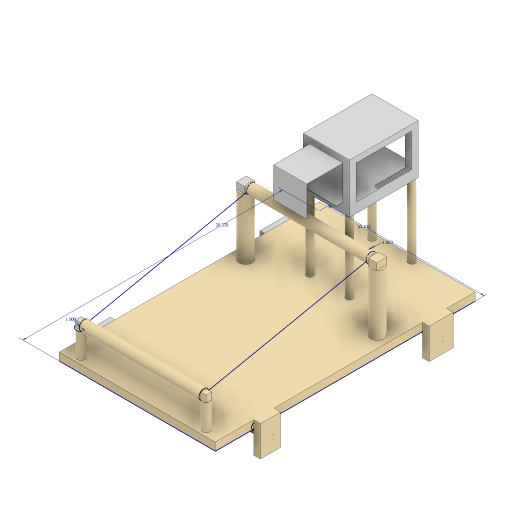
# Autodesk Inventor part: neha_chassis
Saved by Autodesk Inventor 2024 (Build 280153000, 153)
## iProperties
Created: 2023-06-06
Part Number: neha_chassis
Material: Generic
Document SubType Name: Modeling
Designer: ANIRUDH
Density: 1 g/cm^3
Appearance: Default
Author: ANIRUDH
Autodesk Inventor part; units mm, degrees
ref_plane "YZ Plane" through (0, 0, 0) normal (1, 0, 0) x (0, 1, 0)
ref_plane "XZ Plane" through (0, 0, 0) normal (0, 1, 0) x (-1, 0, 0)
sketch "Sketch1" plane through (0, 0, 0) normal (0, 1, 0) x (-1, 0, 0)
  line L0 (-300, -500) -> (300, -500)
  line L1 (300, -500) -> (300, 500)
  line L2 (300, 500) -> (-300, 500)
  line L3 (-300, 500) -> (-300, -500)
  line L4 (-300, -500) -> (300, 500) construction
  line L5 (300, -500) -> (-300, 500) construction
  circle A0 centre (76.2, -479.4561) radius 12.7
  circle A1 centre (-76.2, -479.4561) radius 12.7
  circle A2 centre (76.2, -479.4561) radius 12.7
  point P0 (0, 0)
  dimension "d14" = 600
  dimension "d15" = 1000
  dimension "d24" = 25.4
  constraints: 12 end point, 3 centre point, 2 midpoint, 2 parallel, 1 coincident, 1 concentric, 1 horizontal, 1 perpendicular
  measures "d14" distance of L0.start L0.end
  measures "d15" distance of L0.end L1.end
  measures "d24" diameter of A0
extrude "Extrusion1" add sketch "Sketch1" along normal blind 30 contours L3 L2 L1 L0 | A0 | A1
sketch "Sketch2" plane through (0, 30, 0) normal (0, 1, 0) x (1, 0, 0)
  line L0 (-300, 500) -> (-300, -500) projected
  circle A0 centre (-240.3274, -476.0112) radius 15
  circle A1 centre (241.3, -476.0112) radius 15
  line L1 (300, -500) -> (300, 500) projected
  line L2 (-240.3274, -476.0112) -> (-240.3274, 285.9888)
  line L3 (241.3, -476.0112) -> (241.3, 278.78)
  point P0 (0, 0)
  dimension "d6" = 30
  dimension "d7" = 30
  dimension "d19" = 762
  constraints: 4 end point, 2 centre point, 1 parallel, 1 vertical
  measures "d6" diameter of A0
  measures "d7" diameter of A1
  measures "d19" distance of L2.start L2.end
extrude "Extrusion2" add sketch "Sketch2" along normal blind 100
sketch "Sketch3" plane through (0, 30, 0) normal (0, 1, 0) x (1, 0, 0)
  line L0 (-300, 500) -> (-300, -500) projected
  circle A0 centre (-251.2271, 168.147) radius 25
  circle A1 centre (256.3, 168.147) radius 25
  circle A2 centre (241.3, -476.0112) radius 15 projected
  circle A3 centre (-240.3274, -476.0112) radius 15 projected
  line L1 (269, 155.447) -> (243.6, 180.847) construction
  line L2 (243.6, 155.447) -> (269, 180.847) construction
  point P0 (0, 0)
  dimension "d11" = 50
  dimension "d40" = 25.4
  dimension "d41" = 25.4
  constraints: 4 end point, 2 centre point, 2 midpoint
  measures "d11" diameter of A1
  measures "d40" distance of L1.end L2.end
  measures "d41" distance of L2.start L1.end
extrude "Extrusion3" add sketch "Sketch3" along normal blind 233.807 contours A0 | A1
ref_plane "Work Plane1" through (300, 30, 500) normal (1, 0, 0) x (0, 0, -1)
extrude "Extrusion4" add sketch "Sketch1" along normal blind 309.3974 contours A0 | A1
sketch "Sketch4" plane through (0, 30, 0) normal (0, 1, 0) x (1, 0, 0)
  circle A0 centre (-251.2271, 168.147) radius 25 projected
  circle A1 centre (256.3, 168.147) radius 25 projected
  circle A2 centre (-76.2, 479.4561) radius 12.7 projected
  circle A3 centre (76.2, 479.4561) radius 12.7 projected
  line L0 (76.2, 479.4561) -> (251.876, 479.4561) construction
  circle A4 centre (-76.2, 240.5293) radius 12.7
  circle A5 centre (76.2, 240.5293) radius 12.7
  point P0 (0, 0)
  dimension "d28" = 25.4
  constraints: 2 centre point, 2 end point, 1 horizontal
  measures "d28" diameter of A4
extrude "Extrusion5" add sketch "Sketch4" along normal blind 279.4 contours A4 | A5
sketch "Sketch5" plane through (-76.2, 309.3974, -479.4561) normal (0, 1, 0) x (1, 0, 0)
  line L0 (-14.696, 14.9952) -> (168.2208, 14.9952)
  line L1 (168.2208, 14.9952) -> (168.2208, -255.5835)
  line L2 (168.2208, -255.5835) -> (-14.696, -255.5835)
  line L3 (-14.696, -255.5835) -> (-14.696, 14.9952)
  point P0 (76.2, -479.4561)
  constraints: 8 end point, 2 parallel, 1 horizontal, 1 perpendicular
extrude "Extrusion6" [suppressed]
sketch "Sketch6" plane through (-76.2, 309.3974, -479.4561) normal (0, 1, 0) x (1, 0, 0)
  line L0 (-12.7, 12.7) -> (165.1, 12.7)
  line L1 (165.1, 12.7) -> (165.1, -251.6267)
  line L2 (165.1, -251.6267) -> (-12.7, -251.6267)
  line L3 (-12.7, -251.6267) -> (-12.7, 12.7)
  point P0 (76.2, -479.4561)
  constraints: 8 end point, 2 parallel, 1 horizontal, 1 perpendicular
extrude "Extrusion7" add sketch "Sketch6" along normal blind 12.7
sketch "Sketch7" plane through (300, 0, 500) normal (1, 0, 0) x (0, 0, -1)
  circle A0 centre (149.4368, 9.9643) radius 11.0201
  circle A1 centre (832.4462, 9.9643) radius 9.0585
  point P0 (500, 0)
  constraints: 2 centre point
sketch "Sketch8" plane through (300, 0, 500) normal (1, 0, 0) x (0, 0, -1)
  line L0 (1000, 30) -> (0, 30) projected
  line L1 (148.2506, 30) -> (226.2157, 30)
  line L2 (226.2157, 30) -> (226.2157, -87.9373)
  line L3 (226.2157, -87.9373) -> (148.2506, -87.9373)
  line L4 (148.2506, -87.9373) -> (148.2506, 30)
  line L5 (797.3552, 30) -> (889.8254, 30)
  line L6 (889.8254, 30) -> (889.8254, -87.9373)
  line L7 (889.8254, -87.9373) -> (797.3552, -87.9373)
  line L8 (797.3552, -87.9373) -> (797.3552, 30)
  point P0 (500, 0)
  point P1 (226.2157, 30)
  constraints: 16 end point, 4 parallel, 3 point on line, 2 horizontal, 2 perpendicular
extrude "Extrusion8" add sketch "Sketch8" along normal blind 25.4
sketch "Sketch9" plane through (-300, 0, -500) normal (-1, 0, 0) x (0, 0, 1)
  line L0 (202.6448, -87.9373) -> (110.1746, -87.9373) projected
  line L1 (108.3615, 22.6643) -> (202.6448, 22.6643)
  line L2 (202.6448, 22.6643) -> (202.6448, -87.9373)
  line L3 (202.6448, -87.9373) -> (108.3615, -87.9373)
  line L4 (108.3615, -87.9373) -> (108.3615, 22.6643)
  line L5 (777.4106, 22.6643) -> (851.7494, 22.6643)
  line L6 (851.7494, 22.6643) -> (851.7494, -87.9373)
  line L7 (851.7494, -87.9373) -> (777.4106, -87.9373)
  line L8 (777.4106, -87.9373) -> (777.4106, 22.6643)
  circle A0 centre (142.8112, -48.0482) radius 9.2452
  point P0 (500, 0)
  constraints: 16 end point, 4 parallel, 2 horizontal, 2 perpendicular, 2 point on line, 1 centre point
extrude "Extrusion9" add sketch "Sketch9" along normal blind 25.4 contours L0 L3 L4 L1 L2 | L5 L6 L7 L8 | A0
sketch "Sketch10" plane through (-325.4, 0, -500) normal (-1, 0, 0) x (0, 0, 1)
  circle A0 centre (151.8769, -29.9168) radius 8.1086
  circle A1 centre (802.7946, -29.9168) radius 7.2526
  point P0 (500, 0)
  constraints: 2 centre point
hole "Hole1" at (-325.4, -29.9168, -348.1231) at (-325.4, -29.9168, 302.7946) direction (1, 0, 0) diameter 1.4249 end through all thread size "1-64 UNC" class "2B" standard "ANSI Unified Screw Threads"
sketch "Sketch11" plane through (-325.4, 0, -500) normal (-1, 0, 0) x (0, 0, 1)
  circle A0 centre (148.2506, -46.2351) radius 11.6098
  circle A1 centre (802.7946, -46.2351) radius 11.6316
  point P0 (500, 0)
  constraints: 2 centre point
hole "Hole2" at (-325.4, -46.2351, -351.7494) at (-325.4, -46.2351, 302.7946) direction (1, 0, 0) diameter 1.4249 end through all thread size "1-64 UNC" class "2B" standard "ANSI Unified Screw Threads"
sketch "Sketch12" plane through (-325.4, 0, -500) normal (-1, 0, 0) x (0, 0, 1)
  circle A0 centre (151.8769, -29.9168) radius 0.7125 projected
  circle A1 centre (148.2506, -46.2351) radius 0.7125 projected
  circle A2 centre (151.8769, -29.9168) radius 16.7163
  circle A3 centre (813.6734, -46.6332) radius 18.1314
  point P0 (500, 0)
  constraints: 1 centre point, 1 coincident, 3 other
hole "Hole3" at (-325.4, -29.9168, -348.1231) at (-325.4, -46.6332, 313.6734) direction (1, 0, 0) diameter 1.4249 end through all thread size "1-64 UNC" class "2B" standard "ANSI Unified Screw Threads"
sketch "Sketch13" plane through (-251.2271, 263.807, -168.147) normal (0, 1, 0) x (1, 0, 0)
  circle A0 centre (0, 0) radius 25 projected
  line L0 (-16.0914, -19.1329) -> (16.0914, -19.1329)
  line L1 (16.0914, -19.1329) -> (16.0914, 19.1329)
  line L2 (16.0914, 19.1329) -> (-16.0914, 19.1329)
  line L3 (-16.0914, 19.1329) -> (-16.0914, -19.1329)
  line L4 (-16.0914, -19.1329) -> (16.0914, 19.1329) construction
  line L5 (16.0914, -19.1329) -> (-16.0914, 19.1329) construction
  circle A1 centre (507.5271, 0) radius 25 projected
  line L6 (482.5271, 0) -> (507.5271, 0)
  line L7 (491.4357, -19.1329) -> (523.6185, -19.1329)
  line L8 (523.6185, -19.1329) -> (523.6185, 19.1329)
  line L9 (523.6185, 19.1329) -> (491.4357, 19.1329)
  line L10 (491.4357, 19.1329) -> (491.4357, -19.1329)
  line L11 (491.4357, -19.1329) -> (523.6185, 19.1329) construction
  line L12 (523.6185, -19.1329) -> (491.4357, 19.1329) construction
  point P0 (251.2271, -168.147)
  constraints: 26 end point, 4 midpoint, 4 parallel, 3 horizontal, 3 point on circle, 2 perpendicular
extrude "Extrusion10" add sketch "Sketch13" along normal blind 25.4 contours L1 L0 L3 L2 | L8 L7 L10 L9
sketch "Sketch14" plane through (-240.3274, 130, 476.0112) normal (0, 1, 0) x (1, 0, 0)
  circle A0 centre (0, 0) radius 15 projected
  line L0 (-10.6043, -10.6089) -> (10.6043, -10.6089)
  line L1 (10.6043, -10.6089) -> (10.6043, 10.6089)
  line L2 (10.6043, 10.6089) -> (-10.6043, 10.6089)
  line L3 (-10.6043, 10.6089) -> (-10.6043, -10.6089)
  line L4 (-10.6043, -10.6089) -> (10.6043, 10.6089) construction
  line L5 (10.6043, -10.6089) -> (-10.6043, 10.6089) construction
  circle A1 centre (481.6274, 0) radius 15 projected
  line L6 (471.0231, -10.6089) -> (492.2317, -10.6089)
  line L7 (492.2317, -10.6089) -> (492.2317, 10.6089)
  line L8 (492.2317, 10.6089) -> (471.0231, 10.6089)
  line L9 (471.0231, 10.6089) -> (471.0231, -10.6089)
  line L10 (471.0231, -10.6089) -> (492.2317, 10.6089) construction
  line L11 (492.2317, -10.6089) -> (471.0231, 10.6089) construction
  point P0 (240.3274, 476.0112)
  constraints: 24 end point, 4 midpoint, 4 parallel, 2 horizontal, 2 perpendicular, 2 point on circle, 1 point on line
extrude "Extrusion11" add sketch "Sketch14" along normal blind 25.4 contours L1 L0 L3 L2 | L7 L6 L9 L8
sketch "Sketch15" plane through (240.2086, 263.807, -187.2798) normal (-1, 0, 0) x (0, 0, 1)
  line L0 (0, 0) -> (-5.8671, 0) projected
  line L1 (38.2657, 0) -> (0, 0) projected
  line L2 (0, 0) -> (38.2657, 0)
  line L3 (38.2657, 0) -> (19.1329, 0)
  line L4 (0, 0) -> (0, 25.4) projected
  line L5 (0, 12.7) -> (19.1329, 12.7)
  circle A0 centre (19.1329, 12.7) radius 12.7
  line L6 (0, 25.4) -> (38.2657, 25.4) projected
  point P0 (187.2798, -263.807)
  constraints: 6 end point, 2 midpoint, 1 centre point, 1 coincident, 1 collinear, 1 parallel, 1 tangent
extrude "Extrusion12" add sketch "Sketch15" along normal blind 475.3356 contours A0
sketch "Sketch16" plane through (230.6957, 130, 465.4023) normal (-1, 0, 0) x (0, 0, 1)
  line L0 (0, 0) -> (-4.3911, 0) projected
  line L1 (0, 0) -> (10.6089, 0)
  line L2 (21.2178, 0) -> (0, 0) projected
  line L3 (0, 0) -> (0, 25.4) projected
  line L4 (0, 12.7) -> (10.6089, 12.7)
  circle A0 centre (10.6089, 12.7) radius 12.7
  point P0 (-465.4023, -130)
  point P1 (0, 5.7185)
  point P2 (0, 19.6815)
  constraints: 4 end point, 2 midpoint, 1 centre point, 1 coincident, 1 horizontal
extrude "Extrusion13" add sketch "Sketch16" along normal blind 460.4258 contours A0 L3 picked at (15.4252, 13.6762)
sketch "Sketch17" plane through (300, 0, 500) normal (-1, 0, 0) x (0, 0, 1)
  line L0 (-148.2506, -87.9373) -> (-226.2157, -87.9373) projected
  line L1 (-148.2506, -87.9373) -> (-226.2157, -87.9373)
  line L2 (-226.2157, -87.9373) -> (-187.2331, -87.9373)
  line L3 (-148.2506, 0) -> (-226.2157, 0) projected
  line L4 (-226.2157, -87.9373) -> (-226.2157, 0) projected
  line L5 (-226.2157, 0) -> (-226.2157, -87.9373)
  line L6 (-226.2157, -87.9373) -> (-226.2157, -43.9687)
  point P0 (-500, 0)
  constraints: 8 end point, 2 collinear, 2 midpoint
sketch "Sketch18" plane through (-300, 0, -500) normal (1, 0, 0) x (0, 0, -1)
  point P0 (-500, 0)
sketch "Sketch19" plane through (300, 0, 500) normal (-1, 0, 0) x (0, 0, 1)
  circle A0 centre (-186.3266, -46.6332) radius 0.7125 projected
  circle A1 centre (-186.3266, -46.6332) radius 6.35
  point P0 (-500, 0)
  dimension "d75" = 12.7
  constraints: 1 centre point, 1 coincident
  measures "d75" diameter of A1
extrude "Extrusion14" add sketch "Sketch19" along normal blind 599.9988
sketch "Sketch20" plane through (300, 0, 500) normal (-1, 0, 0) x (0, 0, 1)
  line L0 (-797.3552, 30) -> (-797.3552, -87.9373) projected
  line L1 (-797.3552, -87.9373) -> (-889.8254, -87.9373) projected
  line L2 (-797.3552, -87.9373) -> (-889.8254, -87.9373)
  line L3 (-889.8254, -87.9373) -> (-889.8254, 0)
  line L4 (-889.8254, 0) -> (-889.8254, -43.9687)
  line L5 (-797.3552, -87.9373) -> (-889.8254, -87.9373) projected
  line L6 (-889.8254, -87.9373) -> (-843.5903, -87.9373)
  circle A0 centre (-843.5903, -43.9687) radius 6.35
  point P0 (-500, 0)
  dimension "d78" = 12.7
  constraints: 8 end point, 2 midpoint, 1 centre point, 1 collinear, 1 perpendicular
  measures "d78" diameter of A0
extrude "Extrusion15" add sketch "Sketch20" along normal blind 601.98
sketch "Sketch21" plane through (-235.127, 276.507, -168.147) normal (-1, 0, 0) x (0, 0, 1)
  circle A0 centre (0, 0) radius 12.7 projected
  circle A1 centre (0, 0) radius 19.05
  point P0 (168.147, -276.507)
  point P1 (0, -12.7)
  dimension "d81" = 38.1
  constraints: 1 centre point, 1 coincident, 1 vertical alignment
  measures "d81" diameter of A1
extrude "Extrusion16" add sketch "Sketch21" against normal blind 475.3356
sketch "Sketch22" plane through (0, 130, 0) normal (0, 1, 0) x (1, 0, 0)
  circle A0 centre (-240.3274, -476.0112) radius 15 projected
  circle A1 centre (-240.3274, -476.0112) radius 19.05
  point P0 (0, 0)
  dimension "d84" = 38.1
  constraints: 1 centre point, 1 coincident
  measures "d84" diameter of A1
sketch "Sketch23" plane through (-229.7301, 130, 465.4023) normal (-1, 0, 0) x (0, 0, 1)
  arc A0 (21.2178, 5.7185) -> (21.2178, 19.6815) centre (10.6089, 12.7) ccw projected
  circle A1 centre (10.6089, 12.7) radius 19.05
  point P0 (-465.4023, -130)
  dimension "d85" = 38.1
  constraints: 1 centre point, 1 coincident
  measures "d85" diameter of A1
extrude "Extrusion17" cut sketch "Sketch23" against normal blind 460.4258
sketch "Sketch24" plane through (-229.7301, 130, 465.4023) normal (1, 0, 0) x (0, 0, -1)
  line L0 (-21.2178, 0) -> (-21.2178, 25.4) projected
  line L1 (-21.2178, 25.4) -> (-8.5178, 25.4)
  line L2 (-21.2178, 25.4) -> (0, 25.4) projected
  line L3 (-8.5178, 25.4) -> (0, 25.4)
  line L4 (0, 25.4) -> (0, 12.7)
  circle A0 centre (-9.5657, 12.7) radius 19.05
  point P0 (465.4023, -130)
  dimension "d88" = 12.7
  dimension "d89" = 12.7
  dimension "d90" = 38.1
  constraints: 6 end point, 1 centre point, 1 collinear, 1 perpendicular, 1 point on line
  measures "d88" distance of L0.end L1.end
  measures "d89" distance of L2.end L4.end
  measures "d90" diameter of A0
extrude "Extrusion18" add sketch "Sketch24" along normal blind 460.4258
sketch "Sketch25" plane through (-229.7301, 130, 465.4023) normal (-1, 0, 0) x (0, 0, 1)
  arc A0 (21.2248, -2.3655) -> (-0.007, -3.7701) centre (9.5657, 12.7) ccw projected
  circle A1 centre (9.5657, 12.7) radius 19.05
  arc A2 (-619.3502, 133.807) -> (-647.7483, 133.807) centre (-633.5493, 146.507) ccw projected
  circle A3 centre (-633.5493, 146.507) radius 19.05
  line L0 (9.5657, 12.7) -> (-633.5493, 146.507)
  point P0 (-465.4023, -130)
  constraints: 2 centre point, 2 coincident, 2 end point
sketch "Sketch26" plane through (230.6957, 130, 465.4023) normal (1, 0, 0) x (0, 0, -1)
  arc A0 (0, -3.7742) -> (-21.2178, -2.3709) centre (-9.5657, 12.7) ccw projected
  circle A1 centre (-9.5657, 12.7) radius 19.05
  arc A2 (619.3502, 159.207) -> (619.3502, 133.807) centre (633.5493, 146.507) ccw projected
  circle A3 centre (633.5493, 146.507) radius 19.05
  line L0 (633.5493, 146.507) -> (-9.5657, 12.7)
  point P0 (465.4023, -130)
  constraints: 2 centre point, 2 coincident, 2 end point
sketch "Sketch27" plane through (0, 30, 0) normal (0, 1, 0) x (1, 0, 0)
  point P0 (0, 0)
sketch "Sketch28" plane through (-76.2, 322.0974, -479.4561) normal (0, 1, 0) x (1, 0, 0)
  point P0 (76.2, -479.4561)
sketch "Sketch29" plane through (-76.2, 322.0974, -479.4561) normal (0, 1, 0) x (1, 0, 0)
  line L0 (165.1, 12.7) -> (-12.7, 12.7) projected
  line L1 (-12.7, -251.6267) -> (165.1, -251.6267) projected
  line L2 (-12.7, 12.7) -> (165.1, 12.7)
  line L3 (165.1, 12.7) -> (165.1, -251.6267)
  line L4 (165.1, -251.6267) -> (-12.7, -251.6267)
  line L5 (-12.7, -251.6267) -> (-12.7, 12.7)
  point P0 (76.2, -479.4561)
  constraints: 8 end point, 2 parallel, 1 horizontal, 1 perpendicular
extrude "Extrusion19" add sketch "Sketch29" along normal blind 177.8
sketch "Sketch30" plane through (-76.2, 309.3974, -227.8293) normal (0, 0, 1) x (1, 0, 0)
  line L0 (-12.7, 0) -> (-12.7, 190.5) projected
  line L1 (-12.7, 190.5) -> (-12.7, 165.1)
  line L2 (-12.7, 165.1) -> (-12.7, 38.1)
  line L3 (-12.7, 38.1) -> (-12.7, 12.7)
  line L4 (-12.7, 12.7) -> (12.7, 12.7)
  line L5 (165.1, 0) -> (165.1, 190.5) projected
  line L6 (12.7, 12.7) -> (139.7, 12.7)
  line L7 (139.7, 12.7) -> (165.1, 12.7)
  line L8 (165.1, 12.7) -> (76.2, 12.7)
  line L9 (-12.7, 38.1) -> (-12.7, 101.6)
  line L10 (12.7, 38.1) -> (139.7, 38.1)
  line L11 (139.7, 38.1) -> (139.7, 168.2585)
  line L12 (139.7, 168.2585) -> (12.7, 168.2585)
  line L13 (12.7, 168.2585) -> (12.7, 38.1)
  point P0 (76.2, -309.3974)
  dimension "d95" = 25.4
  dimension "d96" = 127
  dimension "d97" = 25.4
  dimension "d98" = 25.4
  dimension "d99" = 127
  dimension "d100" = 25.4
  constraints: 24 end point, 5 point on line, 2 midpoint, 2 parallel, 2 perpendicular, 1 horizontal
  measures "d95" distance of L0.end L1.end
  measures "d96" distance of L1.end L2.end
  measures "d97" distance of L2.end L3.end
  measures "d98" distance of L3.end L4.end
  measures "d99" distance of L4.end L6.end
  measures "d100" distance of L6.end L7.end
extrude "Extrusion20" cut sketch "Sketch30" against normal blind 381
sketch "Sketch31" plane through (88.9, 309.3974, -240.5293) normal (1, 0, 0) x (0, 0, -1)
  line L0 (-12.7, 0) -> (-12.7, 190.5) projected
  line L1 (-12.7, 190.5) -> (-12.7, 165.1)
  line L2 (-12.7, 165.1) -> (-12.7, 12.7)
  line L3 (-12.7, 12.7) -> (-12.7, 38.1)
  line L4 (-12.7, 38.1) -> (12.7, 38.1)
  line L5 (251.6267, 0) -> (251.6267, 190.5) projected
  line L6 (12.7, 38.1) -> (251.6267, 38.1)
  line L7 (251.6267, 38.1) -> (226.2267, 38.1)
  line L8 (-12.7, 168.2585) -> (251.6267, 168.2585) projected
  line L9 (12.7, 38.1) -> (226.2267, 38.1)
  line L10 (226.2267, 38.1) -> (226.2267, 168.2585)
  line L11 (226.2267, 168.2585) -> (12.7, 168.2585)
  line L12 (12.7, 168.2585) -> (12.7, 38.1)
  point P0 (-240.5293, -309.3974)
  point P1 (12.7, 168.2585)
  point P2 (226.2267, 38.1)
  dimension "d103" = 25.4
  dimension "d104" = 152.4
  dimension "d105" = 25.4
  dimension "d106" = 25.4
  dimension "d107" = 25.4
  constraints: 20 end point, 7 point on line, 2 parallel, 2 perpendicular, 1 horizontal
  measures "d103" distance of L0.end L1.end
  measures "d104" distance of L1.end L2.end
  measures "d105" distance of L2.end L3.end
  measures "d106" distance of L3.end L4.end
  measures "d107" distance of L6.end L7.end
extrude "Extrusion21" cut sketch "Sketch31" against normal blind 381 contours L12 L8 L10 L6
sketch "Sketch32" plane through (88.9, 309.3974, -240.5293) normal (1, 0, 0) x (0, 0, -1)
  line L0 (226.2267, 38.1) -> (251.6267, 38.1) projected
  line L1 (226.2267, 38.1) -> (99.2267, 38.1)
  line L2 (12.7, 38.1) -> (226.2267, 38.1) projected
  line L3 (99.2267, 38.1) -> (105.5767, 38.1)
  line L4 (105.5767, 38.1) -> (99.2267, 38.1)
  line L5 (99.2267, 38.1) -> (99.2267, 44.45)
  line L6 (99.2267, 44.45) -> (226.2267, 44.45)
  line L7 (226.2267, 44.45) -> (226.2267, 38.1)
  point P0 (-240.5293, -309.3974)
  dimension "d110" = 127
  dimension "d111" = 6.35
  dimension "d112" = 6.35
  constraints: 12 end point, 3 perpendicular, 2 point on line, 1 collinear
  measures "d110" distance of L0.start L1.end
  measures "d111" distance of L1.end L3.end
  measures "d112" distance of L1.end L5.end
extrude "Extrusion22" add sketch "Sketch32" against normal blind 15.24
sketch "Sketch33" plane through (88.9, 309.3974, -240.5293) normal (1, 0, 0) x (0, 0, -1)
  line L0 (226.2267, 38.1) -> (251.6267, 38.1) projected
  line L1 (226.2267, 38.1) -> (99.2222, 38.1)
  line L2 (99.2222, 38.1) -> (99.2222, 44.45)
  line L3 (99.2222, 44.45) -> (226.2267, 44.45)
  line L4 (226.2267, 44.45) -> (226.2267, 38.1)
  line L5 (99.2222, 38.1) -> (105.5722, 38.1)
  line L6 (105.5722, 38.1) -> (111.9222, 38.1)
  line L7 (111.9222, 38.1) -> (118.2722, 38.1)
  line L8 (118.2722, 38.1) -> (124.6222, 38.1)
  line L9 (124.6222, 38.1) -> (130.9722, 38.1)
  line L10 (130.9722, 38.1) -> (137.3222, 38.1)
  line L11 (137.3222, 38.1) -> (143.6722, 38.1)
  line L12 (143.6722, 38.1) -> (150.0222, 38.1)
  line L13 (150.0222, 38.1) -> (156.3722, 38.1)
  line L14 (156.3722, 38.1) -> (162.7222, 38.1)
  line L15 (162.7222, 38.1) -> (169.0722, 38.1)
  line L16 (169.0722, 38.1) -> (175.4222, 38.1)
  line L17 (175.4222, 38.1) -> (181.7722, 38.1)
  line L18 (181.7722, 38.1) -> (188.1222, 38.1)
  line L19 (188.1222, 38.1) -> (194.4722, 38.1)
  line L20 (194.4722, 38.1) -> (200.8222, 38.1)
  line L21 (200.8222, 38.1) -> (207.1722, 38.1)
  line L22 (207.1722, 38.1) -> (213.5222, 38.1)
  line L23 (213.5222, 38.1) -> (219.8722, 38.1)
  line L24 (219.8722, 38.1) -> (226.2222, 38.1)
  line L25 (226.2222, 38.1) -> (219.8722, 38.1)
  line L26 (219.8722, 38.1) -> (226.2222, 38.1)
  line L27 (99.2222, 44.45) -> (102.3972, 44.45)
  line L28 (108.7472, 44.45) -> (115.0972, 44.45)
  line L29 (121.4472, 44.45) -> (127.7972, 44.45)
  line L30 (134.1472, 44.45) -> (140.4972, 44.45)
  line L31 (146.8472, 44.45) -> (153.1972, 44.45)
  line L32 (159.5472, 44.45) -> (165.8972, 44.45)
  line L33 (172.2472, 44.45) -> (178.5972, 44.45)
  line L34 (99.2267, 44.45) -> (226.2267, 44.45) projected
  line L35 (184.9472, 44.45) -> (191.2972, 44.45)
  line L36 (197.6472, 44.45) -> (203.9972, 44.45)
  line L37 (210.3472, 44.45) -> (216.6972, 44.45)
  line L38 (223.0472, 44.45) -> (219.8722, 38.1)
  line L39 (219.8722, 38.1) -> (216.6972, 44.45)
  line L40 (213.5222, 38.1) -> (216.6972, 44.45)
  line L41 (210.3472, 44.45) -> (213.5222, 38.1)
  line L42 (207.1722, 38.1) -> (210.3472, 44.45)
  line L43 (200.8222, 38.1) -> (203.9972, 44.45)
  line L44 (194.4722, 38.1) -> (197.6472, 44.45)
  line L45 (188.1222, 38.1) -> (191.2972, 44.45)
  line L46 (181.7722, 38.1) -> (184.9472, 44.45)
  line L47 (175.4222, 38.1) -> (178.5972, 44.45)
  line L48 (169.0722, 38.1) -> (172.2472, 44.45)
  line L49 (162.7222, 38.1) -> (165.8972, 44.45)
  line L50 (156.3722, 38.1) -> (159.5472, 44.45)
  line L51 (153.1972, 44.45) -> (150.0222, 38.1)
  line L52 (146.8472, 44.45) -> (143.6722, 38.1)
  line L53 (140.4972, 44.45) -> (137.3222, 38.1)
  line L54 (134.1472, 44.45) -> (130.9722, 38.1)
  line L55 (127.7972, 44.45) -> (124.6222, 38.1)
  line L56 (121.4472, 44.45) -> (118.2722, 38.1)
  line L57 (115.0972, 44.45) -> (111.9222, 38.1)
  line L58 (108.7472, 44.45) -> (105.5722, 38.1)
  line L59 (102.3972, 44.45) -> (99.2222, 38.1)
  line L60 (102.3972, 44.45) -> (105.5722, 38.1)
  line L61 (108.7472, 44.45) -> (111.9222, 38.1)
  line L62 (115.0972, 44.45) -> (118.2722, 38.1)
  line L63 (121.4472, 44.45) -> (124.6222, 38.1)
  line L64 (127.7972, 44.45) -> (130.9722, 38.1)
  line L65 (134.1472, 44.45) -> (137.3222, 38.1)
  line L66 (140.4972, 44.45) -> (143.6722, 38.1)
  line L67 (146.8472, 44.45) -> (150.0222, 38.1)
  line L68 (153.1972, 44.45) -> (156.3722, 38.1)
  line L69 (159.5472, 44.45) -> (162.7222, 38.1)
  line L70 (165.8972, 44.45) -> (169.0722, 38.1)
  line L71 (172.2472, 44.45) -> (175.4222, 38.1)
  line L72 (178.5972, 44.45) -> (181.7722, 38.1)
  line L73 (184.9472, 44.45) -> (188.1222, 38.1)
  line L74 (191.2972, 44.45) -> (194.4722, 38.1)
  line L75 (197.6472, 44.45) -> (200.8222, 38.1)
  line L76 (203.4681, 43.3917) -> (203.9972, 44.45)
  line L77 (203.9972, 44.45) -> (207.1722, 38.1)
  line L78 (223.0472, 44.45) -> (226.2222, 38.1)
  point P0 (-240.5293, -309.3974)
  point P1 (223.0472, 44.45)
  point P2 (223.0472, 44.45)
  point P3 (203.9972, 44.45)
  point P4 (203.9972, 44.45)
  point P5 (210.3472, 44.45)
  point P6 (210.3472, 44.45)
  point P7 (197.6472, 44.45)
  point P8 (197.6472, 44.45)
  point P9 (191.2972, 44.45)
  point P10 (191.2972, 44.45)
  point P11 (184.9472, 44.45)
  point P12 (184.9472, 44.45)
  point P13 (216.6972, 44.45)
  point P14 (216.6972, 44.45)
  dimension "d115" = 6.35
  dimension "d116" = 6.35
  dimension "d117" = 6.35
  dimension "d118" = 6.35
  dimension "d119" = 6.35
  dimension "d120" = 6.35
  dimension "d121" = 6.35
  dimension "d122" = 6.35
  dimension "d123" = 6.35
  dimension "d124" = 6.35
  dimension "d125" = 6.35
  dimension "d126" = 6.35
  dimension "d127" = 6.35
  dimension "d128" = 6.35
  dimension "d129" = 6.35
  dimension "d130" = 6.35
  dimension "d131" = 6.35
  dimension "d132" = 6.35
  dimension "d133" = 6.35
  dimension "d134" = 6.35
  dimension "d135" = 6.35
  constraints: 150 end point, 21 parallel, 3 collinear, 1 point on line, 1 vertical, 47 other
  measures "d115" distance of L2.start L5.end
  measures "d116" distance of L5.end L6.end
  measures "d117" distance of L6.end L7.end
  measures "d118" distance of L7.end L8.end
  measures "d119" distance of L8.end L9.end
  measures "d120" distance of L9.end L10.end
  measures "d121" distance of L10.end L11.end
  measures "d122" distance of L11.end L12.end
  measures "d123" distance of L12.end L13.end
  measures "d124" distance of L13.end L14.end
  measures "d125" distance of L14.end L15.end
  measures "d126" distance of L15.end L16.end
  measures "d127" distance of L16.end L17.end
  measures "d128" distance of L17.end L18.end
  measures "d129" distance of L18.end L19.end
  measures "d130" distance of L19.end L20.end
  measures "d131" distance of L20.end L21.end
  measures "d132" distance of L21.end L22.end
  measures "d133" distance of L22.end L23.end
  measures "d134" distance of L23.end L24.end
  measures "d135" distance of L24.end L23.end
extrude "Extrusion23" cut sketch "Sketch33" against normal blind 15.24 contours L1 L78 L3 L4 | L39 L3 L38 | L41 L3 L40 | L77 L3 L42 | L75 L3 L43 | L74 L3 L44 | L73 L3 L45 | L72 L3 L46 | L71 L3 L47 | L70 L3 L48 | L69 L3 L49 | L68 L3 L50 | L67 L3 L51 | L66 L3 L52 | L65 L3 L53 | L64 L3 L54 | L63 L3 L55 | L62 L3 L56 | L61 L3 L57 | L60 L3 L58 | L2 L3 L59
sketch "Sketch34" plane through (-76.2, 309.3974, -227.8293) normal (0, 0, 1) x (1, 0, 0)
  line L0 (12.7, 38.1) -> (139.7, 38.1)
  line L1 (139.7, 38.1) -> (139.7, 35.56)
  line L2 (139.7, 35.56) -> (12.7, 35.56)
  line L3 (12.7, 35.56) -> (12.7, 38.1)
  point P0 (76.2, -309.3974)
  dimension "d138" = 127
  dimension "d139" = 2.54
  constraints: 8 end point, 2 parallel, 1 horizontal, 1 perpendicular
  measures "d138" distance of L1.end L2.end
  measures "d139" distance of L0.end L1.end
extrude "Extrusion24" add sketch "Sketch34" along normal blind 25.4
sketch "Sketch35" plane through (-76.2, 309.3974, -227.8293) normal (0, 0, 1) x (1, 0, 0)
  line L0 (12.7, 38.1) -> (12.7, 168.2585) projected
  line L1 (12.7, 168.2585) -> (139.7, 168.2585)
  line L2 (139.7, 168.2585) -> (139.7, 165.7185)
  line L3 (139.7, 165.7185) -> (12.7, 165.7185)
  line L4 (12.7, 165.7185) -> (12.7, 168.2585)
  point P0 (76.2, -309.3974)
  point P1 (12.7, 165.7185)
  dimension "d142" = 127
  dimension "d143" = 2.54
  constraints: 8 end point, 2 parallel, 1 horizontal, 1 perpendicular
  measures "d142" distance of L2.end L3.end
  measures "d143" distance of L1.end L2.end
extrude "Extrusion25" add sketch "Sketch35" along normal blind 127
sketch "Sketch36" plane through (-63.5, 477.6559, -227.8293) normal (0, 1, 0) x (1, 0, 0)
  point P0 (63.5, -227.8293)
sketch "Sketch37" plane through (-76.2, 309.3974, -100.8293) normal (0, 0, 1) x (1, 0, 0)
  line L0 (12.7, 168.2585) -> (139.7, 168.2585) projected
  line L1 (12.7, 165.7185) -> (139.7, 165.7185) projected
  line L2 (12.7, 168.2585) -> (139.7, 168.2585)
  line L3 (139.7, 168.2585) -> (139.7, 165.7185)
  line L4 (139.7, 165.7185) -> (12.7, 165.7185)
  line L5 (12.7, 165.7185) -> (12.7, 168.2585)
  point P0 (76.2, -309.3974)
  constraints: 8 end point, 2 parallel, 1 horizontal, 1 perpendicular
extrude "Extrusion26" add sketch "Sketch37" along normal blind 12.7
sketch "Sketch38" plane through (-63.5, 475.1159, -227.8293) normal (0, -1, 0) x (1, 0, 0)
  line L0 (0, 0) -> (0, 139.7) projected
  line L1 (0, 139.7) -> (127, 139.7)
  line L2 (127, 139.7) -> (127, 137.16)
  line L3 (127, 137.16) -> (0, 137.16)
  line L4 (0, 137.16) -> (0, 139.7)
  point P0 (63.5, 227.8293)
  dimension "d148" = 127
  dimension "d149" = 2.54
  constraints: 8 end point, 2 parallel, 1 horizontal, 1 perpendicular
  measures "d148" distance of L2.end L3.end
  measures "d149" distance of L1.end L2.end
extrude "Extrusion27" add sketch "Sketch38" along normal blind 114.3
body "Solid1"
